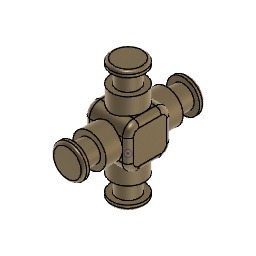
center link v2 (Autodesk Fusion 360 design; units mm, degrees)
Autodesk Fusion 360 part; units mm, degrees
note: some values were not read from the file. Set by a fixed rule: which sketch regions a step uses.
sketch "Sketch1" plane through (0, 0, 0) normal (0, 0, 1) x (1, 0, 0)
sketch "Sketch2" plane through (0, 0, 0) normal (1, 0, 0) x (0, 1, 0)
  circle A0 centre (0, 0) radius 20
  dimension "d4" = 40
  constraint coincident A0.centre origin
  measures "d4" diameter of A0
sketch "Sketch3" plane through (0, 0, 0) normal (0, 0, 1) x (1, 0, 0)
  line L0 (40, -40) -> (-40, -40)
  line L1 (-40, -40) -> (-40, 40)
  line L2 (-40, 40) -> (40, 40)
  line L3 (40, 40) -> (40, -40)
  line L4 (40, -40) -> (-40, 40) construction
  line L5 (-40, -40) -> (40, 40) construction
  dimension "d7" = 80
  dimension "d8" = 80
  constraint horizontal L0
  constraint perpendicular L0 L1
  constraint parallel L0 L2
  constraint parallel L1 L3
  constraint coincident L4 origin
  constraint coincident L5 origin
  measures "d7" distance of L1.end L2.end
  measures "d8" distance of L0.end L1.end
extrude "Extrude2" add sketch "Sketch3" along normal blind 80 makes body 1
sketch "Sketch4" plane through (0, 40, 0) normal (0, 1, 0) x (-1, 0, 0)
  line L0 (-40, 0) -> (40, 0)
  line L1 (40, 0) -> (40, 80)
  line L2 (40, 80) -> (-40, 80)
  line L3 (-40, 80) -> (-40, 0)
  circle A0 centre (0, 40) radius 30
  dimension "d12" = 40
  dimension "d13" = 60
  measures "d12" distance of origin A0.centre
  measures "d13" diameter of A0
extrude "Extrude3" add sketch "Sketch4" along normal blind 30 contours A0 bodies 1
sketch "Sketch5" plane through (0, 0, 80) normal (0, 0, 1) x (-1, 0, 0)
  line L0 (-40, -40) -> (40, -40)
  line L1 (40, -40) -> (40, 40)
  line L2 (40, 40) -> (-40, 40)
  line L3 (-40, 40) -> (-40, -40)
  circle A0 centre (0, 0) radius 30
  dimension "d16" = 60
  constraint coincident A0.centre origin
  measures "d16" diameter of A0
extrude "Extrude4" add sketch "Sketch5" along normal blind 30 contours A0 bodies 1
sketch "Sketch6" plane through (0, 0, 0) normal (0, 0, -1) x (1, 0, 0)
  line L0 (-40, -40) -> (40, -40)
  line L1 (40, -40) -> (40, 40)
  line L2 (40, 40) -> (-40, 40)
  line L3 (-40, 40) -> (-40, -40)
  circle A0 centre (0, 0) radius 30
  dimension "d19" = 60
  constraint coincident A0.centre origin
  measures "d19" diameter of A0
extrude "Extrude5" add sketch "Sketch6" along normal blind 30 contours A0 bodies 1
sketch "Sketch7" plane through (0, -40, 0) normal (0, -1, 0) x (1, 0, 0)
  line L0 (-40, 0) -> (40, 0)
  line L1 (40, 0) -> (40, 80)
  line L2 (40, 80) -> (-40, 80)
  line L3 (-40, 80) -> (-40, 0)
  line L4 (0, 0) -> (0, 40)
  circle A0 centre (0, 40) radius 30
  dimension "d22" = 40
  dimension "d23" = 60
  constraint coincident L4.start origin
  constraint perpendicular L0 L4
  constraint coincident L4.end A0.centre
  measures "d22" distance of L4.start L4.end
  measures "d23" diameter of A0
extrude "Extrude6" add sketch "Sketch7" along normal blind 30 contours A0 bodies 1
sketch "Sketch8" plane through (0, 70, 0) normal (0, 1, 0) x (-1, 0, 0)
  circle A0 centre (0, 40) radius 30
  circle A1 centre (0, 40) radius 20
  dimension "d26" = 40
  dimension "d27" = 40
  measures "d26" distance of origin A0.centre
  measures "d27" diameter of A1
extrude "Extrude7" add sketch "Sketch8" along normal blind 30 contours A1 bodies 1
sketch "Sketch9" plane through (0, 0, 110) normal (0, 0, 1) x (-1, 0, 0)
  circle A0 centre (0, 0) radius 30
  circle A1 centre (0, 0) radius 20
  dimension "d30" = 40
  constraint coincident A0.centre A1.centre
  measures "d30" diameter of A1
extrude "Extrude8" add sketch "Sketch9" along normal blind 30 contours A1 bodies 1
sketch "Sketch10" plane through (0, -70, 0) normal (0, -1, 0) x (1, 0, 0)
  circle A0 centre (0, 40) radius 30
  line L0 (0, 0) -> (0, 40)
  circle A1 centre (0, 40) radius 20
  dimension "d33" = 40
  dimension "d34" = 40
  constraint coincident L0.start origin
  constraint vertical L0
  constraint coincident A0.centre L0.end
  measures "d33" distance of L0.start A0.centre
  measures "d34" diameter of A1
extrude "Extrude9" add sketch "Sketch10" along normal blind 30 contours A1 bodies 1
sketch "Sketch11" plane through (0, 0, -30) normal (0, 0, -1) x (1, 0, 0)
  circle A0 centre (0, 0) radius 30
  circle A1 centre (0, 0) radius 20
  dimension "d37" = 40
  constraint coincident A0.centre A1.centre
  measures "d37" diameter of A1
extrude "Extrude10" add sketch "Sketch11" along normal blind 30 contours A1 bodies 1
fillet "Fillet1" radius 20 1 edges at (0, -40, 80) on bodies 1
fillet "Fillet2" radius 20 3 edges at (0, 40, 80) (0, 40, 0) (0, -40, 0) on bodies 1
fillet "Fillet3" radius 10 16 edges at (40, 40, 40) (40, 34.1421, 5.8579) (40, 0, 0) (40, -34.1421, 5.8579) (40, -40, 40) (40, -34.1421, 74.1421) (40, 0, 80) (40, 34.1421, 74.1421) (-40, -40, 40) (-40, -34.1421, 5.8579) (-40, 0, 0) (-40, 34.1421, 5.8579) (-40, 40, 40) (-40, 34.1421, 74.1421) (-40, 0, 80) (-40, -34.1421, 74.1421) on bodies 1
sketch "Sketch12" plane through (0, 100, 0) normal (0, 1, 0) x (-1, 0, 0)
  circle A0 centre (0, 40) radius 20
  line L0 (0, 0) -> (0, 40)
  circle A1 centre (0, 40) radius 30
  dimension "d46" = 40
  dimension "d47" = 60
  constraint coincident L0.start origin
  constraint vertical L0
  constraint coincident A0.centre L0.end
  measures "d46" distance of L0.start A0.centre
  measures "d47" diameter of A1
extrude "Extrude11" add sketch "Sketch12" along normal blind 10 separate body makes body 2
extrude "Extrude12" add 1 faces at (-0.3664, 100, 45.7735) along direction (0, 1, 0) blind 10 on bodies 1 bodies 1 2
sketch "Sketch13" plane through (0, 0, 140) normal (0, 0, 1) x (-1, 0, 0)
  circle A0 centre (0, 0) radius 20
  circle A1 centre (0, 0) radius 30
  dimension "d52" = 60
  constraint coincident A0.centre A1.centre
  measures "d52" diameter of A1
extrude "Extrude13" add sketch "Sketch13" along normal blind 10 contours A0 | A1 bodies 1
sketch "Sketch14" plane through (0, -100, 0) normal (0, -1, 0) x (1, 0, 0)
  circle A0 centre (0, 40) radius 20
  line L0 (0, 0) -> (0, 40)
  circle A1 centre (0, 40) radius 30
  dimension "d55" = 40
  dimension "d56" = 60
  constraint coincident L0.start origin
  constraint vertical L0
  constraint coincident A0.centre L0.end
  measures "d55" distance of L0.start A0.centre
  measures "d56" diameter of A1
extrude "Extrude14" add sketch "Sketch14" along normal blind 10 contours A0 | A1 bodies 1
sketch "Sketch15" plane through (0, 0, -60) normal (0, 0, -1) x (1, 0, 0)
  circle A0 centre (0, 0) radius 20
  circle A1 centre (0, 0) radius 30
  dimension "d59" = 60
  constraint coincident A0.centre A1.centre
  measures "d59" diameter of A1
extrude "Extrude15" add sketch "Sketch15" along normal blind 10 contours A0 | A1 bodies 1
fillet "Fillet4" radius 5 4 edges at (-27.9698, -110, 29.1515) (-27.9698, 10.8485, -70) (27.9698, 110, 29.1515) (27.9698, 10.8485, 150) on bodies 1
